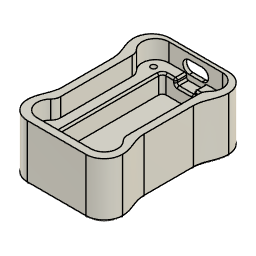
tiny-scarab-enclosure v18 (Autodesk Fusion 360 design; units mm, degrees)
Autodesk Fusion 360 part; units mm, degrees
sketch "Sketch1" plane through (0, 0, 0) normal (0, 0, 1) x (1, 0, 0)
  circle A0 centre (17, 30) radius 3
  circle A1 centre (-17, 30) radius 3
  circle A2 centre (17, -30) radius 3
  circle A3 centre (-17, -30) radius 3
  line L0 (-17.25, 35) -> (-17.25, -35) construction
  line L1 (17.25, 35) -> (17.25, -35) construction
  line L2 (-14.65, 35) -> (-14.65, -35) construction
  line L3 (14.65, 35) -> (14.65, -35) construction
  line L4 (-21, 19.5) -> (21, 19.5) construction
  line L5 (-21, -19.5) -> (21, -19.5) construction
  line L6 (-21, 28.65) -> (21, 28.65) construction
  line L7 (-21, -28.65) -> (21, -28.65) construction
  arc A4 (-14.65, 35) -> (-21, 28.65) centre (-14.65, 28.65) ccw
  arc A5 (21, 28.65) -> (14.65, 35) centre (14.65, 28.65) ccw
  arc A6 (-21, -28.65) -> (-14.65, -35) centre (-14.65, -28.65) ccw
  arc A7 (14.65, -35) -> (21, -28.65) centre (14.65, -28.65) ccw
  line L8 (-14.65, 35) -> (14.65, 35)
  line L9 (-21, 28.65) -> (-21, -28.65) construction
  line L10 (21, 28.65) -> (21, -28.65) construction
  line L11 (19.1082, 26) -> (19.1082, 15) construction
  line L12 (-14.65, -35) -> (14.65, -35)
  line L13 (-19.108, 26.6077) -> (-19.108, 14.6812) construction
  arc A8 (-21, 28.65) -> (-19.108, 24.128) centre (-14.65, 28.65) ccw
  arc A9 (19.1082, 24.1281) -> (21, 28.65) centre (14.65, 28.65) ccw
  line L14 (-19.108, -15) -> (-19.108, -27) construction
  arc A10 (-19.108, -24.128) -> (-21, -28.65) centre (-14.65, -28.65) ccw
  line L15 (19.108, -15.8859) -> (19.108, -24.8859) construction
  arc A11 (21, -28.65) -> (19.108, -24.128) centre (14.65, -28.65) ccw
  arc A12 (19.1082, 24.1281) -> (17.25, 19.5) centre (23.4932, 19.6805) ccw
  arc A13 (-17.25, 19.5) -> (-19.108, 24.128) centre (-23.4921, 19.6809) ccw
  arc A14 (-19.108, -24.128) -> (-17.25, -19.5) centre (-23.4921, -19.6809) ccw
  arc A15 (17.25, -19.5) -> (19.108, -24.128) centre (23.4921, -19.6809) ccw
  line L16 (-17.25, 19.5) -> (-17.25, -19.5)
  line L17 (17.25, 19.5) -> (17.25, -19.5)
  line L18 (0, 35) -> (0, -35) construction
  line L19 (-17.25, 0) -> (17.25, 0) construction
  circle A16 centre (-17, 30) radius 1.5
  circle A17 centre (17, 30) radius 1.5
  circle A18 centre (17, -30) radius 1.5
  circle A19 centre (-17, -30) radius 1.5
  arc A20 (22, 28.65) -> (14.65, 36) centre (14.65, 28.65) ccw
  line L20 (-14.65, 36) -> (14.65, 36)
  arc A21 (-14.65, 36) -> (-22, 28.65) centre (-14.65, 28.65) ccw
  arc A22 (-22, 28.65) -> (-19.81, 23.4158) centre (-14.65, 28.65) ccw
  arc A23 (-18.25, 19.5151) -> (-19.81, 23.4158) centre (-23.4921, 19.6809) ccw
  line L21 (-18.25, 19.5151) -> (-18.25, -19.5151)
  arc A24 (-19.81, -23.4158) -> (-18.25, -19.5151) centre (-23.4921, -19.6809) ccw
  arc A25 (-19.81, -23.4158) -> (-22, -28.65) centre (-14.65, -28.65) ccw
  arc A26 (-22, -28.65) -> (-14.65, -36) centre (-14.65, -28.65) ccw
  line L22 (-14.65, -36) -> (14.65, -36)
  arc A27 (14.65, -36) -> (22, -28.65) centre (14.65, -28.65) ccw
  arc A28 (22, -28.65) -> (19.81, -23.4158) centre (14.65, -28.65) ccw
  arc A29 (18.25, -19.5151) -> (19.81, -23.4158) centre (23.4921, -19.6809) ccw
  line L23 (18.25, 19.5151) -> (18.25, -19.5151)
  arc A30 (19.8102, 23.416) -> (18.25, 19.5151) centre (23.4932, 19.6805) ccw
  arc A31 (19.8102, 23.416) -> (22, 28.65) centre (14.65, 28.65) ccw
  dimension "d3" = 6
  dimension "d7" = 6
  dimension "d8" = 6
  dimension "d9" = 6
  dimension "d25" = 6.35
  dimension "d26" = 6.35
  dimension "d28" = 42
  dimension "d30" = 6.35
  dimension "d31" = 3.75
  dimension "d32" = 70
  dimension "d33" = 60
  dimension "d34" = 6.35
  dimension "d35" = 3.75
  dimension "d36" = 6.35
  dimension "d37" = 15.5
  dimension "d38" = 15.5
  dimension "d39" = 6.35
  dimension "d40" = 1.8918
  dimension "d41" = 1.892
  dimension "d42" = 1.892
  dimension "d43" = 1.892
  dimension "d44" = 34.5
  dimension "d45" = 17.25
  dimension "d46" = 35
  dimension "d48" = 17
  dimension "d50" = 30
  dimension "d51" = 34
  dimension "d52" = 30
  dimension "d53" = 30
  dimension "d56" = 3
  dimension "d58" = 3
  dimension "d59" = 34
  dimension "d60" = 5
  dimension "d61" = 3
  dimension "d62" = 3
  dimension "d83" = -1
  constraint vertical L0
  constraint coincident L2 A4.centre
  constraint coincident L6 A5.centre
  constraint coincident L2 A6.centre
  constraint coincident L7 A6.centre
  constraint coincident L7 A7.centre
  constraint tangent A5 L8
  constraint tangent A7 L10
  constraint perpendicular L4 L11
  constraint tangent A7 L12
  constraint tangent A5 L10
  constraint perpendicular L6 L13
  constraint coincident A4.centre A8.centre
  constraint coincident L13 A8.end
  constraint coincident A5.centre A9.centre
  constraint coincident L11 A9.start
  constraint perpendicular L5 L14
  constraint coincident A6.centre A10.centre
  constraint coincident L14 A10.start
  constraint perpendicular L5 L15
  constraint coincident A7.centre A11.centre
  constraint coincident L15 A11.end
  constraint coincident L4 A12.end
  constraint coincident L1 A12.end
  constraint tangent A9 A12
  constraint coincident L4 A13.start
  constraint coincident L0 A13.start
  constraint tangent A8 A13
  constraint coincident L5 A14.end
  constraint coincident L0 A14.end
  constraint tangent A10 A14
  constraint coincident L1 A15.start
  constraint coincident L5 A15.start
  constraint tangent A11 A15
  constraint vertical L18
  constraint coincident L8 L18.start
  constraint coincident L0 L19.start
  constraint coincident L17 L19.end
  constraint horizontal L19
  constraint midpoint L19 origin
  constraint concentric A1 A16
  constraint concentric A0 A17
  constraint concentric A2 A18
  constraint concentric A3 A19
  measures "d3" diameter of A0
  measures "d7" diameter of A1
  measures "d8" diameter of A3
  measures "d9" diameter of A2
  measures "d25" radius of A4
  measures "d26" radius of A5
  measures "d28" distance of L9 L10
  measures "d30" distance of L3 L10
  measures "d31" distance of L1 L10
  measures "d32" distance of L8 L12
  measures "d33" distance of A0.centre A2.centre
  measures "d34" distance of L2 L9
  measures "d35" distance of L0 L9
  measures "d36" distance of L6 L8
  measures "d37" distance of L4 L8
  measures "d38" distance of L5 L12
  measures "d39" distance of L7 L12
  measures "d40" distance of L10 L11
  measures "d41" distance of L9 L13
  measures "d42" distance of L9 L14
  measures "d43" distance of L10 L15
  measures "d44" distance of L16 L17
  measures "d45" distance of L17 L18
  measures "d46" distance of L12 L19
  measures "d48" distance of A1.centre L18
  measures "d50" distance of A2.centre L19
  measures "d51" distance of A2.centre A3.centre
  measures "d52" distance of A3.centre L19
  measures "d53" distance of A1.centre L19
  measures "d56" diameter of A16
  measures "d58" diameter of A17
  measures "d59" distance of A0.centre A1.centre
  measures "d60" distance of L8 A0.centre
  measures "d61" diameter of A18
  measures "d62" diameter of A19
sketch "weight_cutout_sketch" plane through (0, 0, 0) normal (0, 0, 1) x (1, 0, 0)
  line L0 (-10.25, 30) -> (10.25, 30)
  line L1 (12.25, 28) -> (12.25, -28)
  line L2 (10.25, -30) -> (-10.25, -30)
  line L3 (-12.25, -28) -> (-12.25, 28)
  line L4 (-14.65, 35) -> (14.65, 35)
  line L5 (17.25, 19.5) -> (17.25, -19.5)
  line L6 (-17.25, 19.5) -> (-17.25, -19.5)
  line L7 (-14.65, -35) -> (14.65, -35)
  arc A0 (-10.25, 30) -> (-12.25, 28) centre (-10.25, 28) ccw
  arc A1 (12.25, 28) -> (10.25, 30) centre (10.25, 28) ccw
  arc A2 (-12.25, -28) -> (-10.25, -30) centre (-10.25, -28) ccw
  arc A3 (10.25, -30) -> (12.25, -28) centre (10.25, -28) ccw
  dimension "d63" = 5
  dimension "d64" = 5
  dimension "d65" = 5
  dimension "d66" = 5
  dimension "d67" = 2
  dimension "d68" = 2
  dimension "d69" = 2
  dimension "d70" = 2
  constraint horizontal L0
  constraint vertical L1
  constraint horizontal L2
  constraint vertical L3
  constraint tangent L3 A0
  constraint tangent L0 A0
  constraint tangent L0 A1
  constraint tangent L1 A1
  constraint tangent L3 A2
  constraint tangent L2 A2
  constraint tangent L1 A3
  constraint tangent L2 A3
  measures "d63" distance of L0 L4
  measures "d64" distance of L1 L5
  measures "d65" distance of L3 L6
  measures "d66" distance of L2 L7
  measures "d67" radius of A0
  measures "d68" radius of A1
  measures "d69" radius of A2
  measures "d70" radius of A3
sketch "enclosure_sketch" plane through (0, 0, 0) normal (0, 0, 1) x (1, 0, 0)
  line L0 (-16, 38) -> (16, 38)
  line L1 (26, 28) -> (26, -30) construction
  line L2 (16, -40) -> (-16, -40)
  line L3 (-26, -30) -> (-26, 28) construction
  line L4 (-14.65, 35) -> (14.65, 35) construction
  line L5 (-14.65, -35) -> (14.65, -35) construction
  line L6 (-21, 28.65) -> (-21, -28.65) construction
  line L7 (21, 28.65) -> (21, -28.65) construction
  arc A0 (-16, 38) -> (-26, 28) centre (-16, 28) ccw
  line L8 (-22.25, 47.1324) -> (-22.25, -50) construction
  line L9 (-17.25, 19.5) -> (-17.25, -19.5) construction
  line L10 (-31, 12.5) -> (34.5893, 12.5) construction
  line L11 (-21, 19.5) -> (21, 19.5) construction
  line L12 (-31, -14.5) -> (35, -14.5) construction
  line L13 (-21, -19.5) -> (21, -19.5) construction
  line L14 (22.25, 48) -> (22.25, -50) construction
  line L15 (17.25, 19.5) -> (17.25, -19.5) construction
  spline S0 degree 5 poles (-26, 28) (-26, 27.384) (-25.9234, 26.1659) (-25.5791, 24.3802) (-24.7513, 22.0582) (-23.4987, 19.1339) (-22.6709, 16.655) (-22.3266, 14.6469) (-22.25, 13.2289) (-22.25, 12.5) knots 0 0 0 0 0 0 0.2 0.4 0.6 0.8 1 1 1 1 1 1
  line L16 (-22.25, 14) -> (-22.25, 11)
  arc A1 (26, 28) -> (16, 38) centre (16, 28) ccw
  arc A2 (-26, -30) -> (-16, -40) centre (-16, -30) ccw
  arc A3 (16, -40) -> (26, -30) centre (16, -30) ccw
  spline S1 degree 5 poles (26, 28) (26, 27.3471) (25.9234, 26.0581) (25.5791, 24.175) (24.7513, 21.7449) (23.4987, 18.7551) (22.6709, 16.325) (22.3266, 14.4419) (22.25, 13.1529) (22.25, 12.5) knots 0 0 0 0 0 0 0.2 0.4 0.6 0.8 1 1 1 1 1 1
  spline S2 degree 5 poles (-26, -30) (-26, -29.3492) (-25.9234, -28.0633) (-25.5791, -26.1816) (-24.7513, -23.7484) (-23.4987, -20.7516) (-22.6709, -18.3184) (-22.3266, -16.4367) (-22.25, -15.1508) (-22.25, -14.5) knots 0 0 0 0 0 0 0.2 0.4 0.6 0.8 1 1 1 1 1 1
  spline S3 degree 5 poles (26, -30) (26, -29.3492) (25.9234, -28.0633) (25.5791, -26.1816) (24.7513, -23.7484) (23.4987, -20.7516) (22.6709, -18.3184) (22.3266, -16.4367) (22.25, -15.1508) (22.25, -14.5) knots 0 0 0 0 0 0 0.2 0.4 0.6 0.8 1 1 1 1 1 1
  line L17 (-22.25, 12.5) -> (-22.25, -14.5)
  line L18 (22.25, 12.5) -> (22.25, -14.5)
  dimension "d71" = 3
  dimension "d72" = 5
  dimension "d73" = 5
  dimension "d74" = 5
  dimension "d75" = 10
  dimension "d76" = 5
  dimension "d77" = 7
  dimension "d78" = 5
  dimension "d79" = 5
  dimension "d80" = 10
  dimension "d81" = 10
  dimension "d82" = 10
  dimension "d84" = 25.5
  dimension "d85" = 25.5
  constraint horizontal L0
  constraint vertical L1
  constraint horizontal L2
  constraint vertical L3
  constraint tangent L0 A0
  constraint tangent L3 A0
  constraint parallel L3 L8
  constraint horizontal L10
  constraint horizontal L12
  constraint perpendicular L0 L14
  constraint coincident L10 S0.end
  constraint coincident L8 S0.end
  constraint midpoint S0.end L16
  constraint coincident L8 L16.end
  constraint tangent A0 S0
  constraint tangent L0 A1
  constraint tangent L1 A1
  constraint tangent L3 A2
  constraint tangent L2 A2
  constraint tangent L1 A3
  constraint tangent L2 A3
  constraint coincident L10 S1.end
  constraint coincident L14 S1.end
  constraint coincident L12 S2.end
  constraint coincident L8 S2.end
  constraint coincident L12 S3.end
  constraint coincident L14 S3.end
  constraint tangent A1 S1
  constraint tangent A3 S3
  constraint tangent A2 S2
  measures "d71" distance of L0 L4
  measures "d72" distance of L2 L5
  measures "d73" distance of L3 L6
  measures "d74" distance of L1 L7
  measures "d75" radius of A0
  measures "d76" distance of L8 L9
  measures "d77" distance of L10 L11
  measures "d78" distance of L12 L13
  measures "d79" distance of L14 L15
  measures "d80" radius of A1
  measures "d81" radius of A2
  measures "d82" radius of A3
  measures "d84" distance of L2 L12
  measures "d85" distance of L0 L10
extrude "Extrude2" add sketch "enclosure_sketch" along normal blind 30
sketch "board_fit_cutout_sketch" plane through (0, 0, 0) normal (0, 0, 1) x (1, 0, 0)
  line L0 (-14.65, 36) -> (14.65, 36)
  arc A0 (-14.65, 36) -> (-22, 28.65) centre (-14.65, 28.65) ccw
  arc A1 (-22, 28.65) -> (-19.81, 23.4158) centre (-14.65, 28.65) ccw
  arc A2 (-18.25, 19.5151) -> (-19.81, 23.4158) centre (-23.4921, 19.6809) ccw
  line L1 (-18.25, 19.5151) -> (-18.25, -19.5151)
  arc A3 (-19.81, -23.4158) -> (-18.25, -19.5151) centre (-23.4921, -19.6809) ccw
  arc A4 (-19.81, -23.4158) -> (-22, -28.65) centre (-14.65, -28.65) ccw
  arc A5 (-22, -28.65) -> (-14.65, -36) centre (-14.65, -28.65) ccw
  line L2 (-14.65, -36) -> (14.65, -36)
  arc A6 (14.65, -36) -> (22, -28.65) centre (14.65, -28.65) ccw
  arc A7 (22, -28.65) -> (19.81, -23.4158) centre (14.65, -28.65) ccw
  arc A8 (18.25, -19.5151) -> (19.81, -23.4158) centre (23.4921, -19.6809) ccw
  line L3 (18.25, 19.5151) -> (18.25, -19.5151)
  arc A9 (19.8102, 23.416) -> (18.25, 19.5151) centre (23.4932, 19.6805) ccw
  arc A10 (19.8102, 23.416) -> (22, 28.65) centre (14.65, 28.65) ccw
  arc A11 (22, 28.65) -> (14.65, 36) centre (14.65, 28.65) ccw
extrude "Extrude3" cut sketch "board_fit_cutout_sketch" along normal through all from surface at 20
extrude "Extrude4" cut sketch "weight_cutout_sketch" along normal through all from surface at 10
sketch "usb_cutout_sketch" plane through (0, 36, 0) normal (0, -1, 0) x (1, 0, 0)
  line L0 (14.65, 30) -> (-14.65, 30)
  line L1 (-14.65, 30) -> (-14.65, 20)
  line L2 (-14.65, 20) -> (14.65, 20)
  line L3 (14.65, 20) -> (14.65, 30)
  line L4 (16, 0) -> (-16, 0)
  line L5 (-3.5, 20) -> (3.5, 20)
  arc A0 (3.5, 20) -> (3.5, 27) centre (3.5, 23.5) ccw
  line L6 (3.5, 27) -> (-3.5, 27)
  arc A1 (-3.5, 27) -> (-3.5, 20) centre (-3.5, 23.5) ccw
  line L7 (-3.5, 23.5) -> (3.5, 23.5) construction
  line L8 (-7, 32) -> (-7, 17) construction
  line L9 (7, 32) -> (7, 17) construction
  line L10 (0, 32) -> (0, 17) construction
  line L11 (-16, 0) -> (-16, 30)
  line L12 (16, 0) -> (16, 30)
  dimension "d92" = 20
  dimension "d93" = 14
  dimension "d94" = 7
  dimension "d95" = 7
  dimension "d96" = 32
  dimension "d97" = 16
  constraint tangent L5 A0
  constraint tangent A0 L6
  constraint parallel L5 L6
  constraint tangent L6 A1
  constraint tangent L5 A1
  constraint parallel L0 L7
  constraint vertical L8
  constraint vertical L9
  constraint tangent A0 L9
  constraint tangent A1 L8
  constraint vertical L10
  constraint collinear L2 L5
  measures "d92" distance of L2 L4
  measures "d93" distance of L8 L9
  measures "d94" distance of L5 L6
  measures "d95" distance of L9 L10
  measures "d96" distance of L11 L12
  measures "d97" distance of L10 L12
extrude "Extrude5" cut sketch "usb_cutout_sketch" against normal up to surface (2 mm away) contours L2 L5 A0 L6 A1
sketch "usb_bottom_cutout_sketch" plane through (0, 0, 20) normal (0, 0, 1) x (-1, 0, 0)
  line L0 (-12.25, -28) -> (-12.25, 28)
  arc A0 (-10.25, 30) -> (-12.25, 28) centre (-10.25, 28) ccw
  line L1 (-10.25, 30) -> (10.25, 30)
  arc A1 (12.25, 28) -> (10.25, 30) centre (10.25, 28) ccw
  line L2 (12.25, 28) -> (12.25, -28)
  arc A2 (10.25, -30) -> (12.25, -28) centre (10.25, -28) ccw
  line L3 (10.25, -30) -> (-10.25, -30)
  arc A3 (-12.25, -28) -> (-10.25, -30) centre (-10.25, -28) ccw
  arc A4 (-19.8102, -23.416) -> (-14.65, -36) centre (-14.65, -28.65) ccw
  line L4 (-14.65, -36) -> (-3.5, -36)
  line L5 (-3.5, -36) -> (-3.5, -38)
  line L6 (-3.5, -38) -> (3.5, -38)
  line L7 (3.5, -38) -> (3.5, -36)
  line L8 (3.5, -36) -> (14.65, -36)
  arc A5 (14.65, -36) -> (19.81, -23.4158) centre (14.65, -28.65) ccw
  arc A6 (18.25, -19.5151) -> (19.81, -23.4158) centre (23.4921, -19.6809) ccw
  line L9 (18.25, -19.5151) -> (18.25, 19.5151)
  arc A7 (19.81, 23.4158) -> (18.25, 19.5151) centre (23.4921, 19.6809) ccw
  arc A8 (19.81, 23.4158) -> (14.65, 36) centre (14.65, 28.65) ccw
  line L10 (14.65, 36) -> (-14.65, 36)
  arc A9 (-14.65, 36) -> (-19.81, 23.4158) centre (-14.65, 28.65) ccw
  arc A10 (-18.25, 19.5151) -> (-19.81, 23.4158) centre (-23.4921, 19.6809) ccw
  line L11 (-18.25, 19.5151) -> (-18.25, -19.5151)
  arc A11 (-19.8102, -23.416) -> (-18.25, -19.5151) centre (-23.4932, -19.6805) ccw
  line L12 (5, -36) -> (-5, -36)
  line L13 (-5, -36) -> (-5, -30)
  line L14 (-5, -30) -> (5, -30)
  line L15 (5, -30) -> (5, -36)
  dimension "d100" = 10
  dimension "d101" = 6
  dimension "d102" = 5
  dimension "d103" = 5
  constraint horizontal L12
  constraint vertical L13
  constraint horizontal L14
  constraint vertical L15
  constraint collinear L8 L12
  constraint collinear L3 L14
  measures "d100" distance of L13 L15
  measures "d101" distance of L12 L14
  measures "d102" distance of origin L15
  measures "d103" distance of origin L13
extrude "Extrude6" cut sketch "usb_bottom_cutout_sketch" against normal blind 3 contours L3 L4 L8 L12 L13 L14 L15
fillet "Fillet1" radius 1 1 edges at (-5, 33, 20)
fillet "Fillet2" radius 1 1 edges at (5, 33, 20)
fillet "Fillet3" radius 1 1 edges at (5, 33, 17)
fillet "Fillet4" radius 1 1 edges at (-5, 33, 17)
sketch "Sketch10" plane through (0, 0, 20) normal (0, 0, 1) x (-1, 0, 0)
  line L0 (-6, -36) -> (-6, -30)
  line L1 (-6, -30) -> (-10.25, -30)
  arc A0 (-12.25, -28) -> (-10.25, -30) centre (-10.25, -28) ccw
  line L2 (-12.25, -28) -> (-12.25, 28)
  arc A1 (-10.25, 30) -> (-12.25, 28) centre (-10.25, 28) ccw
  line L3 (-10.25, 30) -> (10.25, 30)
  arc A2 (12.25, 28) -> (10.25, 30) centre (10.25, 28) ccw
  line L4 (12.25, 28) -> (12.25, -28)
  arc A3 (10.25, -30) -> (12.25, -28) centre (10.25, -28) ccw
  line L5 (10.25, -30) -> (6, -30)
  line L6 (6, -30) -> (6, -36)
  line L7 (6, -36) -> (14.65, -36)
  arc A4 (14.65, -36) -> (19.81, -23.4158) centre (14.65, -28.65) ccw
  arc A5 (18.25, -19.5151) -> (19.81, -23.4158) centre (23.4921, -19.6809) ccw
  line L8 (18.25, -19.5151) -> (18.25, 19.5151)
  arc A6 (19.81, 23.4158) -> (18.25, 19.5151) centre (23.4921, 19.6809) ccw
  arc A7 (19.81, 23.4158) -> (14.65, 36) centre (14.65, 28.65) ccw
  line L9 (14.65, 36) -> (-14.65, 36)
  arc A8 (-14.65, 36) -> (-19.81, 23.4158) centre (-14.65, 28.65) ccw
  arc A9 (-18.25, 19.5151) -> (-19.81, 23.4158) centre (-23.4921, 19.6809) ccw
  line L10 (-18.25, 19.5151) -> (-18.25, -19.5151)
  arc A10 (-19.8102, -23.416) -> (-18.25, -19.5151) centre (-23.4932, -19.6805) ccw
  arc A11 (-19.8102, -23.416) -> (-14.65, -36) centre (-14.65, -28.65) ccw
  line L11 (-14.65, -36) -> (-6, -36)
  circle A12 centre (17, -30) radius 1.5
  circle A13 centre (-17, -30) radius 1.5
  circle A14 centre (17, 30) radius 1.5
  circle A15 centre (-17, 30) radius 1.5
extrude "Extrude7" cut sketch "Sketch10" against normal up to surface (20 mm away) contours A12 | A13 | A14 | A15
extrude "Extrude8" cut sketch "board_fit_cutout_sketch" along normal blind 5
fillet "Fillet5" radius 1 12 edges at (0, -40, 0) (23.0711, -37.0711, 0) (24.125, -22.25, 0) (22.25, -1, 0) (24.125, 20.25, 0) (23.0711, 35.0711, 0) (0, 38, 0) (-23.0711, 35.0711, 0) (-24.125, 20.5838, 0) (-22.25, -1, 0) (-24.125, -22.25, 0) (-23.0711, -37.0711, 0)
fillet "Fillet6" radius 1 16 edges at (0, -30, 20) (-11.6642, -29.4142, 20) (-12.25, 0, 20) (-11.6642, 29.4142, 20) (-8.125, 30, 20) (-5.2929, 30, 19.7071) (-5, 30, 18.5) (-4.7071, 30, 17.2929) (0, 30, 17) (4.7071, 30, 17.2929) (5, 30, 18.5) (5.2929, 30, 19.7071) (8.125, 30, 20) (11.6642, 29.4142, 20) (12.25, 0, 20) (11.6642, -29.4142, 20)
